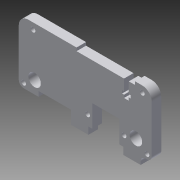
# Autodesk Inventor part: XcrRight_c
Saved by Autodesk Inventor 2013 (Build 170138000, 138)
## iProperties
Created: 2015-01-14
Part Number: XcrRight_c
Material: Generic
Document SubType Name: Modeling
Designer: dzban
Density: 1 g/cm^3
Author: dzban
Autodesk Inventor part; units mm, degrees
ref_plane "YZ Plane" through (0, 0, 0) normal (1, 0, 0) x (0, 1, 0)
ref_plane "XZ Plane" through (0, 0, 0) normal (0, 1, 0) x (-1, 0, 0)
ref_plane "XY Plane" through (0, 0, 0) normal (0, 0, 1) x (1, 0, 0)
sketch "Sketch1" plane through (0, 0, 0) normal (0, 1, 0) x (-1, 0, 0)
  arc A0 (-35.6796, 30.9903) -> (-41.6796, 24.9903) centre (-35.6796, 24.9903) ccw
  line L0 (-41.6796, -5.0097) -> (-41.6796, 24.9903)
  arc A1 (-41.6796, -5.0097) -> (-38.6796, -8.0097) centre (-38.6796, -5.0097) ccw
  line L1 (-37.6796, -8.0097) -> (-38.6796, -8.0097)
  arc A2 (-34.6796, -11.0097) -> (-37.6796, -8.0097) centre (-37.6796, -11.0097) ccw
  line L2 (-34.6796, -13.0097) -> (-34.6796, -11.0097)
  line L3 (-23.6796, -13.0097) -> (-34.6796, -13.0097)
  line L4 (-23.6796, -8.5097) -> (-23.6796, -13.0097)
  line L5 (-21.1796, -8.5097) -> (-23.6796, -8.5097)
  line L6 (-21.1796, 5.4903) -> (-21.1796, -8.5097)
  line L7 (-4.1796, 5.4903) -> (-21.1796, 5.4903)
  line L8 (-4.1796, -8.5097) -> (-4.1796, 5.4903)
  line L9 (-1.6796, -8.5097) -> (-4.1796, -8.5097)
  line L10 (-1.6796, -13.0097) -> (-1.6796, -8.5097)
  line L11 (9.3204, -13.0097) -> (-1.6796, -13.0097)
  line L12 (9.3204, -4.8097) -> (9.3204, -13.0097)
  line L13 (29.8204, -4.8097) -> (9.3204, -4.8097)
  line L14 (29.8204, -8.0097) -> (29.8204, -4.8097)
  line L15 (39.3204, -8.0097) -> (29.8204, -8.0097)
  arc A3 (39.3204, -8.0097) -> (42.3204, -5.0097) centre (39.3204, -5.0097) ccw
  line L16 (42.3204, 24.9903) -> (42.3204, -5.0097)
  arc A4 (42.3204, 24.9903) -> (36.3204, 30.9903) centre (36.3204, 24.9903) ccw
  line L17 (5.8204, 30.9903) -> (36.3204, 30.9903)
  line L18 (5.8204, 28.9903) -> (5.8204, 30.9903)
  line L19 (-24.1796, 28.9903) -> (5.8204, 28.9903)
  line L20 (-24.1796, 21.9903) -> (-24.1796, 28.9903)
  line L21 (-22.9296, 21.9903) -> (-24.1796, 21.9903)
  line L22 (-22.9296, 20.1903) -> (-22.9296, 21.9903)
  line L23 (-24.1796, 20.1903) -> (-22.9296, 20.1903)
  line L24 (-24.1796, 18.3903) -> (-24.1796, 20.1903)
  line L25 (-27.1796, 18.3903) -> (-24.1796, 18.3903)
  line L26 (-27.1796, 20.1903) -> (-27.1796, 18.3903)
  line L27 (-28.4296, 20.1903) -> (-27.1796, 20.1903)
  line L28 (-28.4296, 21.9903) -> (-28.4296, 20.1903)
  line L29 (-27.1796, 21.9903) -> (-28.4296, 21.9903)
  line L30 (-27.1796, 28.9903) -> (-27.1796, 21.9903)
  line L31 (-31.1796, 28.9903) -> (-27.1796, 28.9903)
  line L32 (-31.1796, 30.9903) -> (-31.1796, 28.9903)
  line L33 (-35.6796, 30.9903) -> (-31.1796, 30.9903)
  circle A5 centre (-31.6796, -0.0097) radius 3.96
  circle A6 centre (32.3204, -0.0097) radius 3.96
  circle A7 centre (-35.6796, 26.9903) radius 1.5
  circle A8 centre (-38.6796, -5.0097) radius 1.5
  circle A9 centre (-1.1796, -2.0097) radius 1.5
  circle A10 centre (-24.1796, -2.0097) radius 1.5
  circle A11 centre (33.3204, 26.9903) radius 1.5
  circle A12 centre (39.3204, -5.0097) radius 1.5
  point P0 (0, 0)
  point P1 (0, 0)
  constraints: 68 end point, 13 centre point, 10 point on circle
extrude "Extrusion1" add sketch "Sketch1" along normal blind 6
body "Solid1"
